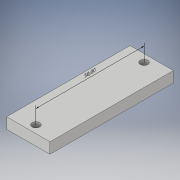
# Autodesk Inventor part: MotorClamp
Saved by Autodesk Inventor 2019 (Build 230136000, 136)
## iProperties
Created: 2018-06-26
Part Number: MotorClamp
Material: Ogólny
Document SubType Name: Modeling
Designer: Kamil
Density: 1 g/cm^3
Appearance: Domyślna
Author: Kamil
Autodesk Inventor part; units mm, degrees
ref_plane "YZ Plane" through (0, 0, 0) normal (1, 0, 0) x (0, 1, 0)
ref_plane "XZ Plane" through (0, 0, 0) normal (0, 1, 0) x (-1, 0, 0)
ref_plane "XY Plane" through (0, 0, 0) normal (0, 0, 1) x (1, 0, 0)
sketch "Szkic1" plane through (0, 0, 0) normal (0, 1, 0) x (-1, 0, 0)
  line L0 (-10, 28.5) -> (10, 28.5)
  line L1 (10, 28.5) -> (10, -28.5)
  line L2 (10, -28.5) -> (-10, -28.5)
  line L3 (-10, -28.5) -> (-10, 28.5)
  line L4 (-10, 28.5) -> (10, -28.5) construction
  line L5 (10, 28.5) -> (-10, -28.5) construction
  circle A0 centre (0, 25) radius 1.75
  circle A1 centre (0, -25) radius 1.75
  point P0 (0, 0)
  dimension "d0" = 20
  dimension "d1" = 57
  dimension "d2" = 3.5
  dimension "d3" = 3.5
  constraints: 12 end point, 2 centre point, 2 midpoint, 2 parallel, 1 horizontal, 1 perpendicular
  measures "d0" distance of L1.end L2.end
  measures "d1" distance of L0.end L1.end
  measures "d2" diameter of A0
  measures "d3" diameter of A1
extrude "Wyciągnięcie proste1" add sketch "Szkic1" along normal blind 5
